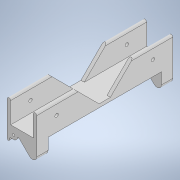
# Autodesk Inventor part: LCD Mount 1
Saved by Autodesk Inventor 2022 (Build 260153000, 153)
## iProperties
Created: 2022-04-02
Part Number: LCD Mount 1
Material: Generic
Document SubType Name: Modeling
Designer: Nick
Density: 1 g/cm^3
Appearance: Default
Author: Nick
Autodesk Inventor part; units mm, degrees
ref_plane "YZ Plane" through (0, 0, 0) normal (1, 0, 0) x (0, 1, 0)
sketch "Sketch2" plane through (0, 0, 0) normal (0, 0, 1) x (1, 0, 0)
  line L0 (3, 23) -> (3, 3)
  line L1 (3, 3) -> (23, 3)
  line L2 (23, 3) -> (23, 23)
  line L3 (2, -7) -> (2, 0)
  line L4 (0, 23) -> (3, 23)
  line L5 (23, 23) -> (26, 23)
  line L6 (26, 23) -> (26, 0)
  line L7 (26, 0) -> (0, 0)
  line L8 (2, -7) -> (9, -7)
  line L9 (9, -7) -> (9, 0)
  line L10 (0, 0) -> (0, 23)
  dimension "d5" = 3
  dimension "d6" = 3
  dimension "d7" = 20
  dimension "d8" = 20
  dimension "d12" = 7
  dimension "d13" = 7
  dimension "d23" = 2
  constraints: 22 end point, 4 vertical, 3 horizontal, 2 collinear, 2 parallel, 2 perpendicular, 2 point on line, 1 coincident
  measures "d5" distance of L2.end L5.end
  measures "d6" distance between parallel lines of L7 L1
  measures "d7" distance of L0.end L1.end
  measures "d8" distance of L1.end L2.end
  measures "d12" distance of L3.start L8.end
  measures "d13" distance of L8.end L9.end
  measures "d23" distance between parallel lines of L10 L3
extrude "Extrusion2" add sketch "Sketch2" along normal blind 120
sketch "Sketch3" plane through (0, 0, 120) normal (0, 0, 1) x (1, 0, 0)
  circle A0 centre (5.5, -3.5) radius 1
  line L0 (2, 0) -> (2, -7) construction
  line L1 (2, -7) -> (9, -7) construction
  point P0 (0, 0)
  point P1 (2, -3.5)
  point P2 (5.5, -7)
  dimension "d17" = 2
  constraints: 2 midpoint, 1 centre point, 1 horizontal alignment, 1 vertical alignment
  measures "d17" diameter of A0
extrude "Extrusion3" cut sketch "Sketch3" against normal through all
ref_plane "Work Plane1" through (0, 0, 60) normal (0, 0, 1) x (1, 0, 0)
sketch "Sketch4" plane through (0, 0, 60) normal (0, 0, 1) x (1, 0, 0)
  circle A0 centre (5.5, -3.5) radius 1 projected
  line L0 (9, -7) -> (9, 0) projected
  line L1 (9, 0) -> (26, 0) projected
  line L2 (26, 0) -> (26, 23) projected
  line L3 (26, 23) -> (23, 23) projected
  line L4 (23, 23) -> (23, 3) projected
  line L5 (23, 3) -> (3, 3) projected
  line L6 (3, 3) -> (3, 23) projected
  line L7 (3, 23) -> (0, 23) projected
  line L8 (2, 0) -> (2, -7) projected
  line L9 (9, -3.5) -> (9, 0) projected
  line L10 (9, 0) -> (0, 0)
  line L11 (0, 23) -> (0, 0) projected
  line L12 (0, 0) -> (2, 0) projected
  line L13 (2, -7) -> (9, -7) projected
  constraints: 2 end point, 1 horizontal
extrude "Extrusion4" cut sketch "Sketch4" along normal mid plane 50 contours L13 L8 L10 L0
fillet "Fillet2" radius 1.5 4 edges at (0, 23, 60) (3, 23, 60) (23, 23, 60) (26, 23, 60)
sketch "Sketch5" plane through (0, 0, 120) normal (0, 0, 1) x (1, 0, 0)
  circle A0 centre (5.5, -3.5) radius 1 projected
  arc A1 (26, 21.5) -> (23, 21.5) centre (24.5, 21.5) ccw projected
  line L0 (23, 21.5) -> (23, 3) projected
  line L1 (23, 3) -> (3, 3) projected
  line L2 (3, 3) -> (3, 21.5) projected
  arc A2 (3, 21.5) -> (0, 21.5) centre (1.5, 21.5) ccw projected
  line L3 (0, 21.5) -> (0, 0) projected
  line L4 (0, 0) -> (2, 0) projected
  line L5 (2, 0) -> (2, -7) projected
  line L6 (2, -7) -> (9, -7) projected
  line L7 (9, -7) -> (9, 0) projected
  line L8 (9, 0) -> (26, 0) projected
  line L9 (26, 0) -> (26, 21.5) projected
  line L10 (0, 0) -> (2, 0) projected
  line L11 (0, 0) -> (2, 0)
  line L12 (2, 0) -> (2, -10)
  line L13 (2, -10) -> (0, -10)
  line L14 (0, -10) -> (0, 0)
  dimension "d24" = 3
  constraints: 8 end point, 2 parallel, 1 collinear, 1 horizontal, 1 perpendicular
  measures "d24" distance between parallel lines of L6 L13
extrude "Extrusion5" add sketch "Sketch5" against normal up to surface (120 mm away) contours L12 L13 L14 L4 L5
fillet "Fillet3" radius 3.5 2 edges at (9, -7, 17.5) (9, -7, 102.5)
fillet "Fillet4" radius 1 2 edges at (0, -10, 60) (2, -10, 60)
sketch "Sketch6" plane through (0, 0, 120) normal (0, 0, 1) x (1, 0, 0)
  line L0 (9, 0) -> (26, 0) projected
  line L1 (9, -2.1213) -> (26, -19.1213)
  line L2 (26, -19.1213) -> (26, 0)
  line L3 (9, -3.5) -> (9, 0) projected
  line L4 (9, 0) -> (12.1001, -3.1001) construction
  point P0 (0, 0)
  dimension "d30" = 45
  dimension "d33" = 45
  dimension "d34" = 1.5
  constraints: 6 end point, 1 perpendicular, 1 point on line
  measures "d30" angle of L0 L1
  measures "d33" angle of L0 L4
  measures "d34" distance from line of L1 L4.end
extrude "Extrusion6" add sketch "Sketch6" against normal blind 10
fillet "Fillet6" radius 3.75 1 edges at (26, -19.1213, 115)
sketch "Sketch7" plane through (9, -2.1213, 120) normal (-0.7071068, -0.7071068, 0) x (-0.7071068, 0.7071068, 0)
  circle A0 centre (-7.4942, 5) radius 3
  line L0 (-14.9883, 0) -> (-14.9883, 10) projected
  line L1 (0, 0) -> (-14.9883, 0) projected
  line L2 (0, 10) -> (0, 0) projected
  line L3 (-14.9883, 10) -> (0, 10) projected
  point P0 (7.864, 120)
  point P1 (-14.9883, 5)
  point P2 (-7.4942, 0)
  dimension "d36" = 6
  constraints: 2 midpoint, 1 centre point, 1 horizontal alignment, 1 vertical alignment
  measures "d36" diameter of A0
extrude "Extrusion7" cut sketch "Sketch7" against normal blind 6 contours A0
chamfer "Chamfer1" distance 0.5 angle 45 1 edges at (16.4205, -9.5418, 115)
fillet "Fillet7" radius 1 1 edges at (9, -2.1213, 115)
ref_plane "Work Plane2" through (0, 0, 60) normal (0, 0, 1) x (1, 0, 0)
mirror "Mirror1" about plane through (0, 0, 60) normal (0, 0, 1) of "Extrusion6", "Fillet6", "Extrusion7", "Chamfer1", "Fillet7"
fillet "Fillet5" radius 1 4 edges at (2, -7, 102.5) (9, 0, 97.5) (2, -7, 17.5) (9, 0, 22.5)
sketch "Sketch8" plane through (26, 21.5, 120) normal (1, 0, 0) x (0, 0, -1)
  line L0 (120, -18.5) -> (0, -18.5) projected
  line L1 (120, -18.5) -> (0, -18.5) projected
  line L2 (120, -18.5) -> (0, -18.5) projected
  line L3 (35, 13.9962) -> (85, 13.9962)
  line L4 (85, 13.9962) -> (85, -18.5)
  line L5 (85, -18.5) -> (35, -18.5)
  line L6 (35, -18.5) -> (35, 13.9962)
  line L7 (0, -31.568) -> (0, 0) projected
  line L8 (120, -31.568) -> (120, 0) projected
  point P0 (120, -21.5)
  point P1 (35, -18.5)
  point P2 (85, -18.5)
  dimension "d43" = 35
  dimension "d44" = 35
  constraints: 8 end point, 2 parallel, 1 horizontal, 1 perpendicular, 1 point on line
  measures "d43" distance between parallel lines of L7 L6
  measures "d44" distance between parallel lines of L8 L4
extrude "Extrusion8" cut sketch "Sketch8" against normal through all
sketch "Sketch9" plane through (26, -10.068, 120) normal (1, 0, 0) x (0, 0, -1)
  line L0 (120, 13.068) -> (85, 13.068) projected
  line L1 (120, 13.068) -> (85, 13.068) projected
  line L2 (35, 13.068) -> (85, 13.068) projected
  line L3 (35, 13.068) -> (0, 13.068) projected
  line L4 (35, 13.068) -> (0, 13.068) projected
  line L5 (85, 13.068) -> (35, 13.068) projected
  line L6 (35, 33.068) -> (0, 33.068) projected
  line L7 (120, 33.068) -> (85, 33.068) projected
  line L8 (85, 33.068) -> (85, 13.068) construction
  line L9 (85, 31.568) -> (85, 33.068) construction
  point P0 (120, 10.068)
  point P1 (17.5, 23.068)
  point P2 (102.5, 23.068)
  point P3 (102.5, 33.068)
  point P4 (85, 23.068)
  point P5 (17.5, 33.068)
  constraints: 3 midpoint, 2 end point, 2 horizontal alignment, 2 vertical alignment, 1 collinear
hole "Hole1" at (26, 13, 102.5) at (26, 13, 17.5) direction (-1, 0, 0) diameter 3 end through all
chamfer "Chamfer2" distance 19.999 angle 45 4 edges at (24.5, 3, 35) (1.5, 3, 35) (1.5, 3, 85) (24.5, 3, 85)
equation "\"d6\" = d5"
body "Solid2"
